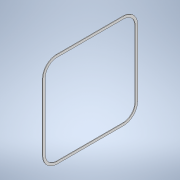
# Autodesk Inventor part: Деталь1
Saved by Autodesk Inventor 2020 (Build 240168000, 168)
## iProperties
Created: 2024-03-28
Part Number: Деталь1
Material: Типовые
Document SubType Name: Modeling
Designer: 4s
Density: 1 g/cm^3
Appearance: По умолчанию
Author: 4s
Autodesk Inventor part; units mm, degrees
ref_plane "YZ Plane" through (0, 0, 0) normal (1, 0, 0) x (0, 1, 0)
ref_plane "XZ Plane" through (0, 0, 0) normal (0, 1, 0) x (-1, 0, 0)
ref_plane "XY Plane" through (0, 0, 0) normal (0, 0, 1) x (1, 0, 0)
sketch "Эскиз1" plane through (0, 0, 0) normal (1, 0, 0) x (0, 1, 0)
  line L0 (10.0569, 70.7059) -> (-130.6091, 70.7059)
  line L1 (-160.6091, 40.7059) -> (-160.6091, -99.9601)
  line L2 (-130.6091, -129.9601) -> (10.0569, -129.9601)
  line L3 (40.0569, -99.9601) -> (40.0569, 40.7059)
  arc A0 (40.0569, 40.7059) -> (10.0569, 70.7059) centre (10.0569, 40.7059) ccw
  arc A1 (10.0569, -129.9601) -> (40.0569, -99.9601) centre (10.0569, -99.9601) ccw
  arc A2 (-160.6091, -99.9601) -> (-130.6091, -129.9601) centre (-130.6091, -99.9601) ccw
  arc A3 (-130.6091, 70.7059) -> (-160.6091, 40.7059) centre (-130.6091, 40.7059) ccw
  point P0 (0, 0)
  point P1 (-160.6091, -129.9601)
  point P2 (-160.6091, 70.7059)
  point P3 (40.0569, -129.9601)
  dimension "d0" = 200.666
  dimension "d1" = 200.666
  dimension "d2" = 30
  constraints: 8 end point, 8 point on circle, 8 tangent, 6 point on line, 4 centre point, 3 equal radius, 2 parallel, 1 horizontal, 1 perpendicular
  measures "d0" distance of point (40.057, -129.96) point (-160.609, -129.96)
  measures "d1" distance of point (-160.609, -129.96) point (-160.609, 70.706)
  measures "d2" radius of A0
extrude "Выдавливание1" add sketch "Эскиз1" along normal blind 1.2
sketch "Эскиз2" plane through (1.2, 0, 0) normal (1, 0, 0) x (0, 0, -1)
  line L0 (-40.7059, -160.6091) -> (99.9601, -160.6091) projected
  arc A0 (99.9601, -160.6091) -> (129.9601, -130.6091) centre (99.9601, -130.6091) ccw projected
  line L1 (129.9601, -130.6091) -> (129.9601, 10.0569) projected
  arc A1 (129.9601, 10.0569) -> (99.9601, 40.0569) centre (99.9601, 10.0569) ccw projected
  line L2 (99.9601, 40.0569) -> (-40.7059, 40.0569) projected
  arc A2 (-40.7059, 40.0569) -> (-70.7059, 10.0569) centre (-40.7059, 10.0569) ccw projected
  line L3 (-70.7059, 10.0569) -> (-70.7059, -130.6091) projected
  arc A3 (-70.7059, -130.6091) -> (-40.7059, -160.6091) centre (-40.7059, -130.6091) ccw projected
  line L4 (-40.7059, 35.0569) -> (99.9601, 35.0569)
  arc A4 (124.9601, 10.0569) -> (99.9601, 35.0569) centre (99.9601, 10.0569) ccw
  line L5 (124.9601, 10.0569) -> (124.9601, -130.6091)
  arc A5 (99.9601, -155.6091) -> (124.9601, -130.6091) centre (99.9601, -130.6091) ccw
  line L6 (99.9601, -155.6091) -> (-40.7059, -155.6091)
  arc A6 (-65.7059, -130.6091) -> (-40.7059, -155.6091) centre (-40.7059, -130.6091) ccw
  line L7 (-65.7059, -130.6091) -> (-65.7059, 10.0569)
  arc A7 (-40.7059, 35.0569) -> (-65.7059, 10.0569) centre (-40.7059, 10.0569) ccw
  point P0 (0, 0)
  dimension "d5" = 5
  constraints: 8 end point, 8 point on circle, 4 centre point, 7 other
  measures "d5" distance between parallel lines of L2 L4
extrude "Выдавливание2" cut sketch "Эскиз2" against normal up to surface (1.2 mm away) contours L4 A4 L5 A5 L6 A6 L7 A7
